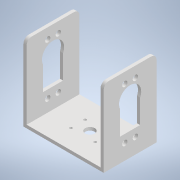
# Autodesk Inventor part: 7
Saved by Autodesk Inventor 2021 (Build 250183000, 183)
## iProperties
Created: 2021-03-30
Part Number: 7
Material: Genérico
Document SubType Name: Modeling
Designer: diego
Density: 1 g/cm^3
Appearance: Valor por defecto
Author: diego
Autodesk Inventor part; units mm, degrees
ref_plane "YZ Plane" through (0, 0, 0) normal (1, 0, 0) x (0, 1, 0)
ref_plane "XZ Plane" through (0, 0, 0) normal (0, 1, 0) x (-1, 0, 0)
ref_plane "XY Plane" through (0, 0, 0) normal (0, 0, 1) x (1, 0, 0)
sketch "Boceto1" plane through (0, 0, 0) normal (0, 0, 1) x (1, 0, 0)
  line L0 (0, 0) -> (76, 0)
  line L1 (76, 0) -> (76, 73)
  line L2 (76, 73) -> (73, 73)
  line L3 (73, 73) -> (73, 3)
  line L4 (73, 3) -> (3, 3)
  line L5 (3, 3) -> (3, 73)
  line L6 (3, 73) -> (0, 73)
  line L7 (0, 73) -> (0, 0)
  constraints: 16 end point, 2 horizontal, 2 parallel, 2 perpendicular, 2 point on line, 1 vertical
extrude "Extrusión1" add sketch "Boceto1" against normal blind 50
sketch "Boceto2" plane through (76, 0, 0) normal (1, 0, 0) x (0, 0, -1)
  circle A0 centre (25, 49) radius 6.5
  circle A1 centre (20, 63) radius 2.5
  circle A2 centre (30, 63) radius 2.5
  circle A3 centre (20, 14.5) radius 2.5
  circle A4 centre (30, 14.5) radius 2.5
  point P0 (0, 0)
  point P1 (0, 73)
  constraints: 5 centre point
hole "Agujero1" at (76, 63, -20) at (76, 63, -30) at (76, 14.5, -20) at (76, 14.5, -30) direction (-1, 0, 0) diameter 5 end through all
hole "Agujero2" at (76, 49, -25) direction (-1, 0, 0) diameter 13 end through all
sketch "Boceto3" plane through (3, 3, 0) normal (0, 1, 0) x (1, 0, 0)
  circle A0 centre (35, 25) radius 4.5
  circle A1 centre (46.5, 31.75) radius 1.25
  circle A2 centre (46.5, 18.25) radius 1.25
  circle A3 centre (23.5, 31.75) radius 1.25
  circle A4 centre (23.5, 18.25) radius 1.25
  constraints: 5 centre point
hole "Agujero3" at (38, 3, -25) direction (0, -1, 0) diameter 9 end through all
hole "Agujero4" at (26.5, 3, -18.25) at (26.5, 3, -31.75) at (49.5, 3, -31.75) at (49.5, 3, -18.25) direction (0, -1, 0) diameter 2.5 end through all
fillet "Empalme1" radius 5 4 edges at (1.5, 73, 0) (1.5, 73, -50) (74.5, 73, 0) (74.5, 73, -50)
sketch "Boceto4" plane through (76, 0, 0) normal (1, 0, 0) x (0, 0, -1)
  circle A0 centre (25, 49) radius 6.5 projected
  arc A1 (34.5, 44.5279) -> (15.5, 44.5279) centre (25, 49) ccw
  line L0 (25, 22) -> (34.5, 22)
  line L1 (34.5, 22) -> (34.5, 44.5279)
  line L2 (25, 22) -> (15.5, 22)
  line L3 (15.5, 22) -> (15.5, 44.5279)
  point P0 (0, 0)
  dimension "d68" = 9.5
  dimension "d69" = 9.5
  constraints: 8 end point, 2 perpendicular, 2 point on circle, 1 centre point, 1 coincident, 1 point on line
  measures "d68" distance of L0.start L0.end
  measures "d69" distance of L0.start L2.end
extrude "Extrusión2" cut sketch "Boceto4" against normal blind 100 contours A0 | L1 L0 L2 L3 A1
